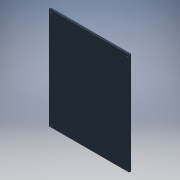
# Autodesk Inventor part: M178-2005
Saved by Autodesk Inventor 2018 (Build 220105000, 105)
## iProperties
Created: 2004-11-20
Part Number: M178-2005
Document SubType Name: Modeling
Designer: Autodesk, Inc.
Manufacturer: Standard
Standards Organization: Custom
Description: CABINET, PC, BASE PANEL
Mass: 1728.74 g
Surface Area: 3801.39 cm^2
Volume: 1728.74 cm^3
Density: 1 g/cm^3
Material: Generic
Appearance: Blue Gray (Dark/Polished)
CAGE: 1LJX3
Dept. ID: Product Design
Description #2: ---
Finish #1: ---
Finish #2: ---
Material ID: ---
Project Number: ---
Author: Autodesk, Inc.
Autodesk Inventor part; units mm, degrees
ref_plane "YZ Plane" through (0, 0, 0) normal (1, 0, 0) x (0, 1, 0)
ref_plane "XZ Plane" through (0, 0, 0) normal (0, 1, 0) x (-1, 0, 0)
ref_plane "XY Plane" through (0, 0, 0) normal (0, 0, 1) x (1, 0, 0)
sketch "Sketch1" plane through (0, 0, 0) normal (0, 0, 1) x (1, 0, 0)
  line L0 (-189.23, 240.03) -> (189.23, 240.03)
  line L1 (189.23, 240.03) -> (189.23, -240.03)
  line L2 (189.23, -240.03) -> (-189.23, -240.03)
  line L3 (-189.23, -240.03) -> (-189.23, 240.03)
  point P0 (0, 0)
  point P1 (-189.23, 0)
  point P2 (0, 240.03)
  dimension "d0" = 378.46
  dimension "d1" = 480.06
  constraints: 8 end point, 2 midpoint, 2 parallel, 1 horizontal, 1 horizontal alignment, 1 perpendicular, 1 vertical alignment
  measures "d0" distance of L0.start L0.end
  measures "d1" distance of L2.end L0.start
extrude "Extrusion1" add sketch "Sketch1" along normal blind 9.525
sketch "Sketch2" plane through (0, 0, 9.525) normal (0, 0, 1) x (1, 0, 0)
  line L0 (189.23, -240.03) -> (-189.23, -240.03) projected
  line L1 (189.23, 240.03) -> (189.23, -240.03) projected
  point P0 (180.5, -231.3)
  dimension "d4" = 8.73
  dimension "d5" = 8.73
  measures "d4" distance from line of L0 point (180.5, -231.3)
  measures "d5" distance from line of point (180.5, -231.3) L1
hole "Hole1" at (180.5, -231.3, 9.525) direction (0, 0, -1) diameter 6.604 end through all countersink diameter 12.5984 countersink angle 90 clearance for "Flat Head Machine Screw" size "M6" standard "Ansi Metric M Profile"
mirror "Mirror1" about plane through (0, 0, 0) normal (0, 1, 0) of "Hole1"
mirror "Mirror2" about plane through (0, 0, 0) normal (1, 0, 0) of "Hole1", "Mirror1"
body "Solid1"
